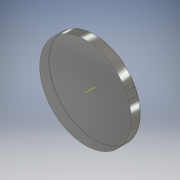
# Autodesk Inventor part: Mirror
Saved by Autodesk Inventor 2019.4 (Build 234330000, 330)
## iProperties
Created: 2019-05-26
Part Number: Mirror
Material: Szkło
Document SubType Name: Modeling
Designer: barto
Density: 2.18 g/cm^3
Appearance: Przezroczyste
Author: barto
Autodesk Inventor part; units mm, degrees
ref_plane "YZ Plane" through (0, 0, 0) normal (1, 0, 0) x (0, 1, 0)
ref_plane "XZ Plane" through (0, 0, 0) normal (0, 1, 0) x (-1, 0, 0)
ref_plane "XY Plane" through (0, 0, 0) normal (0, 0, 1) x (1, 0, 0)
sketch "Szkic2" plane through (0, 0, 0) normal (1, 0, 0) x (0, 1, 0)
  line L0 (-15.4661, 0) -> (-15.4661, -100)
  line L1 (-15.4661, -100) -> (4.5339, -100)
  arc A0 (0, 0) -> (4.5339, -98.5) centre (999.9945, -3.3247) ccw
  line L2 (4.5339, -100) -> (4.5339, -98.5)
  line L3 (0, 0) -> (-15.4661, 0)
  line L4 (-218.5582, 0) -> (1203.0866, 0) projected
  dimension "d1" = 1000
  dimension "d6" = 1.5
  dimension "d7" = 20
  dimension "d9" = 100
  constraints: 8 end point, 3 point on circle, 2 vertical, 1 centre point, 1 horizontal, 1 perpendicular
  measures "d1" radius of A0
  measures "d6" distance of L2.end L1.end
  measures "d7" distance of L0.end L1.end
  measures "d9" distance of L0.start L0.end
revolve "Obrót1" add sketch "Szkic2" angle 360 about axis through (0, -10, 0) along (0, 1, 0)
